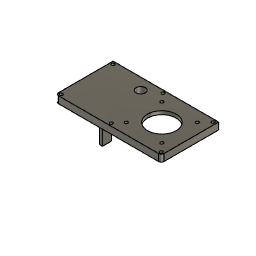
LidV2 (Autodesk Fusion 360 design; units mm, degrees)
Autodesk Fusion 360 part; units mm, degrees
note: some values were not read from the file. Set by a fixed rule: the direction of a hole.
sketch "Sketch33" plane through (0, 0, 0) normal (0, 0, 1) x (1, 0, 0)
  line L0 (58, -25) -> (-34, -25)
  line L1 (-34, -25) -> (-34, 25)
  line L2 (-34, 25) -> (58, 25)
  line L3 (58, 25) -> (58, -25)
  circle A0 centre (33.55, 0) radius 12.5
  circle A1 centre (0, 15) radius 4
  circle A2 centre (49.05, 15.5) radius 1.325
  circle A3 centre (49.05, -15.5) radius 1.325
  circle A4 centre (18.05, 15.5) radius 1.325
  circle A5 centre (18.05, -15.5) radius 1.325
  circle A6 centre (-31.621, -22.621) radius 1.3375
  circle A7 centre (-31.621, -22.621) radius 2.379
  circle A8 centre (12, -22.621) radius 1.3375
  circle A9 centre (12, -22.621) radius 2.379
  circle A10 centre (55.621, -22.621) radius 1.3375
  circle A11 centre (55.621, -22.621) radius 2.379
  circle A12 centre (-31.621, 22.621) radius 1.3375
  circle A13 centre (-31.621, 22.621) radius 2.379
  circle A14 centre (12, 22.621) radius 1.3375
  circle A15 centre (12, 22.621) radius 2.379
  circle A16 centre (55.621, 22.621) radius 1.3375
  circle A17 centre (55.621, 22.621) radius 2.379
  circle A18 centre (0, 15) radius 5
  dimension "d258" = 92
  dimension "d259" = 50
  dimension "d260" = 25
  dimension "d261" = 24.45
  dimension "d262" = 25
  dimension "d263" = 8
  dimension "d265" = 34
  dimension "d275" = 2.65
  dimension "d278" = 31
  dimension "d279" = 31
  dimension "d280" = 2.675
  dimension "d281" = 2.379
  dimension "d282" = 2.379
  dimension "d285" = 87.242
  dimension "d286" = 45.242
  dimension "d324" = 15
  constraint horizontal L0
  constraint vertical L1
  constraint horizontal L2
  constraint vertical L3
  constraint concentric A6 A7
  constraint tangent L0 A7
  constraint concentric A1 A18
  measures "d258" distance of L1.end L2.end
  measures "d259" distance of L0.end L1.end
  measures "d260" diameter of A0
  measures "d261" distance of L3 A0.centre
  measures "d262" distance of L2 A0.centre
  measures "d263" diameter of A1
  measures "d265" distance of L1 A1.centre
  measures "d275" diameter of A2
  measures "d280" diameter of A6
  measures "d281" distance of L0 A6.centre
  measures "d282" distance of L1 A6.centre
  measures "d324" distance of origin A1.centre
extrude "Extrude1" add sketch "Sketch33" along normal blind 6 contours L0 L3 A11 | A15 | A9 | L0 L1 L2 L3 A7 A11 A13 A17 | A11 | L2 L3 A17 | A17 | L0 L1 A7 | A7 | L1 L2 A13 | A13 | A6 | A8 | A10 | A12 | A14 | A16 | A18
shell "Shell1" thickness 3 removed faces 7 at (19.3734, -15.566, 4) at (47.8864, 14.8663, 4) at (49.2801, -14.1951, 4) at (46.0345, -0.6231, 4) at (3.995, 14.8006, 4) at (18.595, 16.7077, 4) at (-7.0275, -12.9078, 0)
hole "Hole2" at (55.621, -22.621, 0) at (55.621, 22.621, 0) at (12, -22.621, 0) at (12, 22.621, 0) at (-31.621, -22.621, 0) at (-31.621, 22.621, 0) direction (0, 0, 1) diameter 2.675 end up to surface (6 mm away)
fillet "Fillet1" radius 2.379 2 edges at (58, -25, 3) (-34, -25, 3)
sketch "Sketch5" plane through (0, 0, 0) normal (0, 0, -1) x (1, 0, 0)
  line L0 (-30.4364, 22) -> (10.8154, 22)
  line L1 (55, 21.4364) -> (55, -21.4364)
  line L2 (54.4364, -22) -> (13.1846, -22)
  line L3 (-31, -21.4364) -> (-31, 21.4364)
  arc A0 (-31.621, 25) -> (-34, 22.621) centre (-31.621, 22.621) ccw
  line L4 (-34, 22.621) -> (-34, -25)
  line L5 (-34, -25) -> (58, -25)
  line L6 (58, -25) -> (58, 22.621)
  arc A1 (58, 22.621) -> (55.621, 25) centre (55.621, 22.621) ccw
  line L7 (55.621, 25) -> (-31.621, 25)
  arc A2 (-30.4364, 22) -> (-31, 21.4364) centre (-31.621, 22.621) ccw
  arc A3 (13.1846, 22) -> (10.8154, 22) centre (12, 22.621) ccw
  line L8 (13.1846, 22) -> (54.4364, 22)
  arc A4 (55, 21.4364) -> (54.4364, 22) centre (55.621, 22.621) ccw
  arc A5 (54.4364, -22) -> (55, -21.4364) centre (55.621, -22.621) ccw
  arc A6 (10.8154, -22) -> (13.1846, -22) centre (12, -22.621) ccw
  line L9 (10.8154, -22) -> (-30.4364, -22)
  arc A7 (-31, -21.4364) -> (-30.4364, -22) centre (-31.621, -22.621) ccw
  line L10 (55.621, 23.5) -> (-31.621, 23.5)
  arc A8 (-31.621, 23.5) -> (-32.5, 22.621) centre (-31.621, 22.621) ccw
  line L11 (-32.5, 22.621) -> (-32.5, -22.621)
  arc A9 (-32.5, -22.621) -> (-31.621, -23.5) centre (-31.621, -22.621) ccw
  line L12 (-31.621, -23.5) -> (55.621, -23.5)
  arc A10 (55.621, -23.5) -> (56.5, -22.621) centre (55.621, -22.621) ccw
  line L13 (56.5, -22.621) -> (56.5, 22.621)
  arc A11 (56.5, 22.621) -> (55.621, 23.5) centre (55.621, 22.621) ccw
  constraint concentric A0 A8
  constraint concentric A1 A11
  constraint tangent L10 A8
  constraint tangent L10 A11
  constraint tangent A8 L11
  constraint tangent L11 A9
  constraint tangent A9 L12
  constraint tangent L12 A10
  constraint tangent A10 L13
  constraint tangent L13 A11
extrude "Extrude4" cut sketch "Sketch5" against normal blind 1.5 contours L0 A2 A3 L10 | L3 A2 A7 L11 | A3 L8 A4 L10 | A6 L9 A7 L12 | L1 A4 A5 L13 | L2 A5 A6 L12
extrude "Extrude3" add sketch "Sketch33" along normal blind 3 contours A15 | A9 | A11 | A17 | A7 | A13
sketch "Sketch2" plane through (0, 0, 0) normal (0, 0, -1) x (1, 0, 0)
  line L0 (-34, -25) -> (58, -25)
  line L1 (58, -25) -> (58, 22.621)
  arc A0 (58, 22.621) -> (55.621, 25) centre (55.621, 22.621) ccw
  line L2 (55.621, 25) -> (-31.621, 25)
  arc A1 (-31.621, 25) -> (-34, 22.621) centre (-31.621, 22.621) ccw
  line L3 (-34, 22.621) -> (-34, -25)
  arc A2 (47.5013, 17.8933) -> (52, 13.5) centre (52, 18) ccw
  line L4 (-28, 13.5) -> (52, 13.5)
  arc A3 (-28, 13.5) -> (-23.5023, 17.8555) centre (-28, 18) ccw
  line L5 (-24.7584, -21.2368) -> (-23.5023, 17.8555)
  arc A4 (-24.7584, -21.2368) -> (-29.2843, -16.5924) centre (-29.2561, -21.0923) ccw
  line L6 (52.8867, -16.0776) -> (-29.2843, -16.5924)
  arc A5 (52.8867, -16.0776) -> (48.4162, -20.6842) centre (52.9149, -20.5775) ccw
  line L7 (47.5013, 17.8933) -> (48.4162, -20.6842)
  circle A6 centre (-31.621, -22.621) radius 1.3375
  circle A7 centre (12, 22.621) radius 1.3375
  circle A8 centre (55.621, 22.621) radius 1.3375
  circle A9 centre (-31.621, 22.621) radius 1.3375
  circle A10 centre (12, -22.621) radius 1.3375
  arc A11 (-29.4103, -23.5) -> (-32.5, -20.4103) centre (-31.621, -22.621) ccw
  line L8 (-32.5, -20.4103) -> (-32.5, 20.4103)
  arc A12 (-32.5, 20.4103) -> (-29.4103, 23.5) centre (-31.621, 22.621) ccw
  line L9 (-29.4103, 23.5) -> (9.7893, 23.5)
  arc A13 (9.7893, 23.5) -> (14.2107, 23.5) centre (12, 22.621) ccw
  line L10 (14.2107, 23.5) -> (53.4103, 23.5)
  arc A14 (53.4103, 23.5) -> (56.5, 20.4103) centre (55.621, 22.621) ccw
  line L11 (56.5, 20.4103) -> (56.5, -20.4103)
  arc A15 (56.5, -20.4103) -> (53.4103, -23.5) centre (55.621, -22.621) ccw
  line L12 (53.4103, -23.5) -> (14.2107, -23.5)
  arc A16 (14.2107, -23.5) -> (9.7893, -23.5) centre (12, -22.621) ccw
  line L13 (9.7893, -23.5) -> (-29.4103, -23.5)
  circle A17 centre (55.621, -22.621) radius 1.3375
  constraint tangent A2 L7
  constraint tangent L5 A4
  constraint tangent L4 A3
  constraint tangent A2 L4
  constraint tangent A3 L5
  constraint tangent A5 L7
  constraint tangent A4 L6
  constraint tangent L6 A5
extrude "Extrude5" add sketch "Sketch33" against normal blind 3 from surface at 3 contours A18
fillet "Fillet2" radius 2 1 edges at (-4.6616, 13.1919, 3)
sketch "Sketch6" plane through (0, 0, 3) normal (0, 0, -1) x (1, 0, 0)
  circle A0 centre (33.55, 0) radius 12.5
  circle A1 centre (18.05, 15.5) radius 1.325
  circle A2 centre (49.05, 15.5) radius 1.325
  circle A3 centre (49.05, -15.5) radius 1.325
  circle A4 centre (18.05, -15.5) radius 1.325
  arc A5 (-29.3245, -22) -> (-31, -20.3245) centre (-31.621, -22.621) ccw
  line L0 (-29.3245, -22) -> (0, -22)
  circle A6 centre (0, -15) radius 7
  line L1 (0, -22) -> (9.7035, -22)
  arc A7 (14.2965, -22) -> (9.7035, -22) centre (12, -22.621) ccw
  line L2 (14.2965, -22) -> (53.3245, -22)
  arc A8 (55, -20.3245) -> (53.3245, -22) centre (55.621, -22.621) ccw
  line L3 (55, -20.3245) -> (55, 20.3245)
  arc A9 (53.3245, 22) -> (55, 20.3245) centre (55.621, 22.621) ccw
  line L4 (53.3245, 22) -> (14.2965, 22)
  arc A10 (9.7035, 22) -> (14.2965, 22) centre (12, 22.621) ccw
  line L5 (9.7035, 22) -> (-29.3245, 22)
  arc A11 (-31, 20.3245) -> (-29.3245, 22) centre (-31.621, 22.621) ccw
  line L6 (-31, 20.3245) -> (-31, -20.3245)
  line L7 (-4.85, 16) -> (-2.35, 16)
  line L8 (-2.35, 16) -> (-2.35, 8)
  line L9 (-2.35, 8) -> (-4.85, 8)
  line L10 (-4.85, 8) -> (-4.85, 16)
  line L11 (12.65, 7.37) -> (12.65, 16)
  line L12 (-15, -12.75) -> (-15, -15.25)
  line L13 (-15, -15.25) -> (-25, -15.25)
  line L14 (-25, -15.25) -> (-25, -12.75)
  line L15 (-25, -12.75) -> (-15, -12.75)
  line L16 (-15, -12.75) -> (-25, -15.25) construction
  line L17 (-15, -15.25) -> (-25, -12.75) construction
  point P0 (-20, -14)
  dimension "d375" = 8
  dimension "d376" = 6
  dimension "d378" = 15
  dimension "d379" = 2.5
  dimension "d380" = 10
  dimension "d395" = 2.5
  dimension "d396" = 6.75
  dimension "d397" = 6
  constraint horizontal L7
  constraint vertical L8
  constraint horizontal L9
  constraint vertical L10
  constraint perpendicular L12 L13
  constraint parallel L12 L14
  constraint parallel L13 L15
  constraint coincident L16 P0
  constraint coincident L17 P0
  measures "d375" distance of L7.end L8.end
  measures "d376" distance of L5 L7.end
  measures "d378" distance of L8.end L11
  measures "d379" distance of L13.end L14.end
  measures "d380" distance of L12.end L13.end
  measures "d395" distance of L8.end L9.end
  measures "d396" distance of L0 L12.end
  measures "d397" distance of L6 L14.end
extrude "Extrude6" add sketch "Sketch6" along normal blind 35 contours L12 L13 L14 L15
extrude "Extrude7" add sketch "Sketch6" along normal blind 25 contours L7 L8 L9 L10
